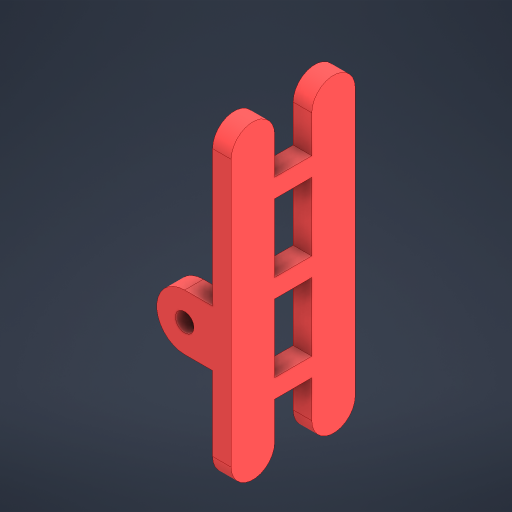
# Autodesk Inventor part: agarre_izquierda
Saved by Autodesk Inventor 2023.1 (Build 271208000, 208)
## iProperties
Created: 2022-10-23
Part Number: agarre_izquierda
Material: Generic
Document SubType Name: Modeling
Designer: amtat
Density: 1 g/cm^3
Appearance: Default
Author: amtat
Autodesk Inventor part; units mm, degrees
ref_plane "YZ Plane" through (0, 0, 0) normal (1, 0, 0) x (0, 1, 0)
ref_plane "XZ Plane" through (0, 0, 0) normal (0, 1, 0) x (-1, 0, 0)
ref_plane "XY Plane" through (0, 0, 0) normal (0, 0, 1) x (1, 0, 0)
sketch "Sketch1" plane through (0, 0, 0) normal (0, 0, 1) x (1, 0, 0)
  circle A0 centre (0, 0) radius 1.5
  circle A1 centre (0, 0) radius 4.5
  line L0 (4.5, 0) -> (4.5, 4.5)
  line L1 (4.5, 4.5) -> (0, 4.5)
  line L2 (4.5, 0) -> (4.5, -4.5)
  line L3 (4.5, -4.5) -> (0, -4.5)
  dimension "d0" = 3
  dimension "d1" = 9
  constraints: 8 end point, 3 point on circle, 2 centre point, 2 coincident, 2 tangent, 1 point on line, 1 vertical
  measures "d0" diameter of A0
  measures "d1" diameter of A1
extrude "Extrusion1" add sketch "Sketch1" along normal blind 3
sketch "Sketch2" plane through (4.5, -4.5, 0) normal (1, 0, 0) x (0, 0, -1)
  line L0 (0, 0) -> (0, 9) projected
  line L1 (0, 9) -> (-3, 9) projected
  line L2 (-3, 0) -> (-3, 9) projected
  line L3 (0, 0) -> (-3, 0) projected
  line L4 (-3, 9) -> (-3, 0) projected
  line L5 (-3, 0) -> (-3, 4.5)
  line L6 (-3, 4.5) -> (-3, 34.5)
  line L7 (-3, 34.5) -> (17, 34.5)
  line L8 (17, 34.5) -> (17, -15.5)
  line L9 (17, -15.5) -> (-3, -15.5)
  line L10 (-3, -15.5) -> (-3, 4.5)
  point P0 (0, 4.5)
  dimension "d4" = 4.5
  dimension "d5" = 30
  dimension "d6" = 20
  dimension "d7" = 50
  constraints: 12 end point, 3 perpendicular, 2 point on line, 1 collinear, 1 midpoint
  measures "d4" distance of L2.start L5.end
  measures "d5" distance of L5.end L6.end
  measures "d6" distance of L6.end L7.end
  measures "d7" distance of L7.end L8.end
extrude "Extrusion2" add sketch "Sketch2" along normal blind 3
sketch "Sketch3" plane through (7.5, -4.5, 0) normal (1, 0, 0) x (0, 0, -1)
  line L0 (-3, -15.5) -> (17, -15.5) projected
  line L1 (17, -15.5) -> (17, 34.5) projected
  line L2 (17, 34.5) -> (-3, 34.5) projected
  line L3 (-3, 34.5) -> (-3, -15.5) projected
  line L4 (-3, 0) -> (-3, -15.5) projected
  line L5 (-3, -15.5) -> (0, -15.5)
  line L6 (-3, -15.5) -> (17, -15.5) projected
  line L7 (0, -15.5) -> (0, 34.5)
  line L8 (17, -15.5) -> (14, -15.5)
  line L9 (14, -15.5) -> (14, 34.5)
  line L10 (17, 34.5) -> (-3, 34.5) projected
  line L11 (0, -15.5) -> (0, 9.5)
  line L12 (0, 9.5) -> (0, 11)
  line L13 (0, 11) -> (14, 11)
  line L14 (14, 11) -> (14, 8)
  line L15 (14, 8) -> (0, 8)
  line L16 (0, 8) -> (0, 9.5)
  line L17 (0, 9.5) -> (0, -4.5)
  line L18 (0, -4.5) -> (0, -6)
  line L19 (0, -6) -> (14, -6)
  line L20 (14, -6) -> (14, -3)
  line L21 (14, -3) -> (0, -3)
  line L22 (0, 9.5) -> (0, 23.5)
  line L23 (0, 23.5) -> (0, 25)
  line L24 (0, 25) -> (14, 25)
  line L25 (14, 25) -> (14, 22)
  line L26 (14, 22) -> (0, 22)
  line L27 (0, -15.5) -> (4, -15.5)
  line L28 (4, -15.5) -> (4, 34.5)
  line L29 (14, -15.5) -> (10, -15.5)
  line L30 (10, -15.5) -> (10, 34.5)
  point P0 (0, 4.5)
  point P1 (10, -6)
  point P2 (4, -6)
  point P3 (10, -3)
  point P4 (10, 8)
  point P5 (4, 8)
  point P6 (4, -3)
  point P7 (10, 11)
  point P8 (10, 22)
  point P9 (4, 22)
  point P10 (4, 11)
  point P11 (10, 25)
  point P12 (4, 25)
  dimension "d10" = 3
  dimension "d11" = 3
  dimension "d12" = 25
  dimension "d13" = 1.5
  dimension "d14" = 3
  dimension "d15" = 14
  dimension "d16" = 1.5
  dimension "d17" = 3
  dimension "d18" = 14
  dimension "d19" = 1.5
  dimension "d20" = 3
  dimension "d21" = 4
  dimension "d22" = 4
  constraints: 48 end point, 22 point on line, 10 perpendicular, 1 collinear, 1 midpoint
  measures "d10" distance of L0.start L5.end
  measures "d11" distance of L0.end L8.end
  measures "d12" distance of L5.end L11.end
  measures "d13" distance of L11.end L12.end
  measures "d14" distance of L13.end L14.end
  measures "d15" distance of L11.end L17.end
  measures "d16" distance of L17.end L18.end
  measures "d17" distance of L19.end L20.end
  measures "d18" distance of L11.end L22.end
  measures "d19" distance of L22.end L23.end
  measures "d20" distance of L24.end L25.end
  measures "d21" distance of L5.end L27.end
  measures "d22" distance of L8.end L29.end
extrude "Extrusion3" cut sketch "Sketch3" against normal blind 3 contours L28 L19 L30 L0 | L28 L15 L30 L21 | L2 L30 L24 L28 | L28 L26 L30 L13
sketch "Sketch4" plane through (7.5, -4.5, 0) normal (1, 0, 0) x (0, 0, -1)
  line L0 (10, -6) -> (10, -15.5) projected
  line L1 (10, -15.5) -> (17, -15.5) projected
  line L2 (17, -15.5) -> (17, 34.5) projected
  line L3 (17, 34.5) -> (10, 34.5) projected
  line L4 (10, 34.5) -> (10, 25) projected
  line L5 (10, 25) -> (4, 25) projected
  line L6 (4, 25) -> (4, 34.5) projected
  line L7 (4, 34.5) -> (-3, 34.5) projected
  line L8 (-3, 34.5) -> (-3, -15.5) projected
  line L9 (-3, -15.5) -> (4, -15.5) projected
  line L10 (4, -15.5) -> (4, -6) projected
  line L11 (4, -6) -> (10, -6) projected
  line L12 (4, -3) -> (4, 8) projected
  line L13 (4, 8) -> (10, 8) projected
  line L14 (10, 8) -> (10, -3) projected
  line L15 (10, -3) -> (4, -3) projected
  line L16 (4, 11) -> (4, 22) projected
  line L17 (4, 22) -> (10, 22) projected
  line L18 (10, 22) -> (10, 11) projected
  line L19 (10, 11) -> (4, 11) projected
  line L20 (-3, -15.5) -> (0.5, -15.5)
  line L21 (-3, -15.5) -> (4, -15.5) projected
  line L22 (0.5, -15.5) -> (0.5, -12)
  circle A0 centre (0.5, -12) radius 3.5
  line L23 (-3, -15.5) -> (-3, 9.5)
  line L24 (-3, 34.5) -> (-3, -15.5) projected
  line L25 (-3, 9.5) -> (5.4894, 9.5)
  circle A1 centre (0.5, 31) radius 3.5
  line L26 (-3, 9.5) -> (7, 9.5)
  line L27 (7, 9.5) -> (7, 17.879)
  circle A2 centre (13.5, -12) radius 3.5
  circle A3 centre (13.5, 31) radius 3.5
  point P0 (0, 4.5)
  point P1 (-3, 31)
  point P2 (0.5, 34.5)
  point P3 (4, 31)
  point P4 (10, 31)
  point P5 (13.5, 34.5)
  point P6 (17, 31)
  point P7 (17, -12)
  point P8 (13.5, -15.5)
  point P9 (10, -12)
  point P10 (-3, -12)
  point P11 (4, -12)
  dimension "d25" = 3.5
  dimension "d26" = 3.5
  dimension "d27" = 25
  constraints: 12 end point, 4 centre point, 3 symmetric about line, 2 midpoint, 2 perpendicular, 1 coincident, 1 horizontal, 1 parallel, 1 tangent, 3 other
  measures "d25" distance of L8.end L20.end
  measures "d26" distance of L20.end L22.end
  measures "d27" distance of L8.end L23.end
extrude "Extrusion4" cut sketch "Sketch4" against normal blind 3 contours A2 L1 L0 | L2 L1 A2 | L10 L9 A0 | A3 L3 L2 | L9 L8 A0 | A3 L4 L3 | L8 L7 A1 | L7 L6 A1
fillet "Fillet1" radius 2 1 edges at (4.5, 0, 0)
body "Solid1"
